# Autodesk Inventor part: 欧标 2020铝合金钢材-01
Saved by Autodesk Inventor 2021 (Build 250183000, 183)
## iProperties
Created: 2025-04-16
Part Number: 欧标 2020铝合金钢材-01
Material: 常规
Document SubType Name: Modeling
Designer: 86155
Standards Organization: GB
Language: zh-CN
Size Designation: 欧标 2020铝合金钢材-01
Categories: <MemberInstance><Categories><Category DisplayName="结构型材" InternalName="089c4875-fa83-4c05-b084-43b9cc11f5ed" Mnemonic="GRDR"><CategoryParameter DisplayName="每单位长度的质量" InternalName="0bb95a10-148f-4027-a459-38d7b056702a" Mnemonic="shpmass"/><CategoryParameter DisplayName="截面面积" InternalName="1ff91680-64b0-4202-b9a3-7fd3f94bba3b" Mnemonic="secarea"/><CategoryParameter DisplayName="旋转半径 (x)" InternalName="25778675-03e9-40c1-b6a8-4a9ed693320d" Mnemonic="gyrradx"/><CategoryParameter DisplayName="扭转刚性模数" InternalName="26c1ec35-5026-4c63-ad0a-751cf684a536" Mnemonic="torrigmod"/><CategoryParameter DisplayName="重心到 X-X 的距离" InternalName="26c9bdb8-9c79-4b4f-a92e-8e197583c9c4" Mnemonic="grcendistX"/><CategoryParameter DisplayName="旧成员 ID" InternalName="340afe4f-75d7-48d3-ab7d-943f3c3da468" Mnemonic="LegacyMemberID"/><CategoryParameter DisplayName="基本长度" InternalName="42e34263-8f20-4d0e-ad48-bf1385b87c24" Mnemonic="shplen"/><CategoryParameter DisplayName="转动惯量 (y)" InternalName="4b9f58ea-bced-460e-81ea-3d29ca5a49e3" Mnemonic="inermomy"/><CategoryParameter DisplayName="转动惯量 (x)" InternalName="4cd780bc-73d7-43ac-917a-579e5cbd684d" Mnemonic="inermomx"/><CategoryParameter DisplayName="自定义基点" InternalName="4f1d1b73-316d-484b-a3df-9cbabb16eb77" Mnemonic="shpBasePoint"/><CategoryParameter DisplayName="形状高度" InternalName="50274e7d-5ac0-4796-92cb-c59e54983c67" Mnemonic="shpheig"/><CategoryParameter DisplayName="截面模数 (y)" InternalName="59eaa5e9-d227-48dc-b6c1-6920f96e0f95" Mnemonic="secmody"/><CategoryParameter DisplayName="截面指示" InternalName="5a64d034-428d-49c8-ba32-7619764de20f" Mnemonic="shpdes"/><CategoryParameter DisplayName="截面模数 (x)" InternalName="72cfad18-cf51-4ed4-aaa7-c6b224f8419f" Mnemonic="secmodx"/><CategoryParameter DisplayName="扭转截面模数" InternalName="7c55a8dc-8844-49f9-a867-cc677b30ec9a" Mnemonic="torsecmod"/><CategoryParameter DisplayName="形状宽度" InternalName="7c717d54-a18f-4666-b4d4-573cce22c62c" Mnemonic="shpwdth"/><CategoryParameter DisplayName="第二个形状厚度" InternalName="9251a8e1-85fd-4e47-af99-afdb762317d9" Mnemonic="shpthick2"/><CategoryParameter DisplayName="编写的 FG" InternalName="9c666724-f362-4ea7-ac62-f6a007de5c69" Mnemonic="shpFGAuto"/><CategoryParameter DisplayName="重心到 Y-Y 的距离" InternalName="bcc4fb17-7af4-436a-8f8c-d0aa3b0248c5" Mnemonic="grcendistY"/><CategoryParameter DisplayName="旋转半径 (y)" InternalName="bfa18ebe-1636-4dbe-8d42-b263e0b73184" Mnemonic="gyrrady"/><CategoryParameter DisplayName="形状厚度" InternalName="d109cf76-8eb4-42fc-9800-4409734adc67" Mnemonic="shpthick"/><CategoryParameter DisplayName="剪切位移系数" InternalName="de4c90c6-aaa8-468f-a335-6737b311b5d3" Mnemonic="shdispc"/><Category DisplayName="其他" InternalName="f02205ff-2390-476f-921c-0b3185f88e84" Mnemonic="OTHSHP"><CategoryParameter DisplayName="转动惯量 (y)" InternalName="044c654e-f649-48ac-84cc-650a29ae31ca" Mnemonic="inermomy"/><CategoryParameter DisplayName="形状厚度" InternalName="12b1a788-9233-48fd-a933-2df8ff42b15f" Mnemonic="shpthick"/><CategoryParameter DisplayName="每单位长度的质量" InternalName="2fd289d6-9394-4d2d-97e6-6659d7d4551d" Mnemonic="shpmass"/><CategoryParameter DisplayName="旋转半径 (y)" InternalName="743e1dfe-1bba-408b-b985-cf752b207386" Mnemonic="gyrrady"/><CategoryParameter DisplayName="截面模数 (y)" InternalName="88b8bff9-a616-4028-93d5-ed4f79680d13" Mnemonic="secmody"/><CategoryParameter DisplayName="截面面积" InternalName="c46ecdf8-b6eb-4db9-8b25-30258930c1e3" Mnemonic="secarea"/><CategoryParameter DisplayName="截面模数 (x)" InternalName="cac70804-9d39-43bb-be17-56ea1f39a6c2" Mnemonic="secmodx"/><CategoryParameter DisplayName="转动惯量 (x)" InternalName="ec6737bc-264f-43ed-b0bd-f6d410c2718d" Mnemonic="inermomx"/><CategoryParameter DisplayName="旋转半径 (x)" InternalName="ee72c61e-565e-4fd6-b448-66e1e1abcb7e" Mnemonic="gyrradx"/></Category></Category><Category DisplayName="数据类型" InternalName="23b78d0f-2648-40c6-8793-ca6db495c9e8" Mnemonic="DATATYPE"><CategoryParameter DisplayName="显示名" InternalName="05415f3d-3907-474b-a020-eb9d644f4cf3" Mnemonic="DISPLAYNAME"/><CategoryParameter DisplayName="标准" InternalName="0c0a119c-1e12-4c84-803f-101930972f5e" Mnemonic="STANDARD"/><CategoryParameter DisplayName="描述" InternalName="13903e3d-64b1-4950-80da-f627842ea37f" Mnemonic="DESCRIPTION"/><CategoryParameter DisplayName="规格" InternalName="2675968c-4ce5-49e0-a4f5-552d29089031" Mnemonic="DESIGNATION"/><CategoryParameter DisplayName="默认列" InternalName="2af9ec52-faaa-4026-b378-f9fa4afca842" Mnemonic="DEFAULTROW"/><CategoryParameter DisplayName="文件夹名称" InternalName="3f06958e-8713-4116-9be7-ed6184ecc97b" Mnemonic="FOLDERNAME"/><CategoryParameter DisplayName="版本指南" InternalName="45a75005-10b1-4dfc-8d6d-dfe629f0b93c" Mnemonic="REVISIONGUID"/><CategoryParameter DisplayName="文件名" InternalName="8b46a4cc-9585-4fed-90c3-899f57e09a73" Mnemonic="FILENAME"/><CategoryParameter DisplayName="标准组织" InternalName="8f5914e1-4693-403f-8ab5-d37768198c9d" Mnemonic="STDSORG"/><CategoryParameter DisplayName="系列版本" InternalName="914462f6-6e19-4b14-ba84-155b9680b1d0" Mnemonic="FAMILYREVISION"/><CategoryParameter DisplayName="标准版本" InternalName="91d5a463-65c2-4fde-b823-3b7fea5e8e17" Mnemonic="STANDARDREVISION"/><CategoryParameter DisplayName="成员版本" InternalName="a65d44b9-392f-4f4f-857b-e4b3d54996fe" Mnemonic="MEMBERREVISION"/><CategoryParameter DisplayName="剪裁格式" InternalName="bc51e27b-3422-4e78-93ef-cec197ddf230" Mnemonic="CLIPFORMAT"/><CategoryParameter DisplayName="制造商" InternalName="cd6c7a72-a28a-4e50-99a9-2c7f4e13e5ad" Mnemonic="MANUFACTURER"/><CategoryParameter DisplayName="内部名称" InternalName="cf1d0246-76d9-4b4a-8305-fa0409afb5c1" Mnemonic="INTERNALNAME"/><CategoryParameter DisplayName="是否公制" InternalName="e2385c5b-1ea4-4823-96a8-8de651266ec3" Mnemonic="ISMETRIC"/><Category DisplayName="零件" InternalName="c0e0b642-3bcb-4cc8-9e80-f96d35c4afa4" Mnemonic="PART"><CategoryParameter DisplayName="零件代号" InternalName="016b6077-bfbe-49bd-92c9-d8d59c39c941" Mnemonic="PARTNUMBER"/><CategoryParameter DisplayName="库存编号" InternalName="4dba7c1c-e26c-444e-836c-b08b433409a8" Mnemonic="STOCKNUMBER"/><CategoryParameter DisplayName="材料键" InternalName="5c9a8adb-dd2b-4535-b97f-0a94a95fe41f" Mnemonic="MATERIALKEY"/><CategoryParameter DisplayName="材料" InternalName="818a152a-d3c3-49ca-80ee-df7d91421b8e" Mnemonic="MATERIAL"/></Category></Category></Categories><FamilyTemplate Id="欧标 2020铝合金钢材"><FamilyTemplateParameters><FamilyTemplateParameter ObjectType="kUserParameterObject" ValueType="xs:double" Id="2" ObjectReferenceKey="圆角"/><FamilyTemplateParameter ObjectType="kUserParameterObject" ValueType="xs:double" Id="3" ObjectReferenceKey="宽度"/><FamilyTemplateParameter ObjectType="kUserParameterObject" ValueType="xs:double" Id="4" ObjectReferenceKey="长度"/><FamilyTemplateParameter ObjectType="kPartComponentDefinitionObject" ValueType="xs:string" Id="6" SubObjectId="Material"/><FamilyTemplateParameter ObjectType="kPropertyObject" ValueType="xs:string" Id="18" ObjectReferenceKey="{32853F0F-3444-11d1-9E93-0060B03C1CA6}" SubObjectId="5"/><FamilyTemplateParameter ObjectType="kPropertyObject" ValueType="xs:string" Id="19" ObjectReferenceKey="{32853F0F-3444-11d1-9E93-0060B03C1CA6}" SubObjectId="52"/></FamilyTemplateParameters></FamilyTemplate><CategoryParameterMap><ParamToTemplateMap><ParamToTemplate CategoryParameter="//CategoryParameter[@InternalName='cf1d0246-76d9-4b4a-8305-fa0409afb5c1']" ConstantValue="f6263a19-3060-40e9-a912-404bc1cf63e0"/><ParamToTemplate CategoryParameter="//CategoryParameter[@InternalName='45a75005-10b1-4dfc-8d6d-dfe629f0b93c']" ConstantValue="6f9f3c90-dcaa-4261-b2d0-a83ec9cae418"/><ParamToTemplate CategoryParameter="//CategoryParameter[@InternalName='3f06958e-8713-4116-9be7-ed6184ecc97b']" ConstantValue="欧标 2020铝合金钢材"/><ParamToTemplate CategoryParameter="//CategoryParameter[@InternalName='8f5914e1-4693-403f-8ab5-d37768198c9d']" ConstantValue="GB"/><ParamToTemplate CategoryParameter="//CategoryParameter[@InternalName='0c0a119c-1e12-4c84-803f-101930972f5e']" TemplateParameter="12"/><ParamToTemplate CategoryParameter="//CategoryParameter[@InternalName='91d5a463-65c2-4fde-b823-3b7fea5e8e17']" TemplateParameter="13"/><ParamToTemplate CategoryParameter="//CategoryParameter[@InternalName='cd6c7a72-a28a-4e50-99a9-2c7f4e13e5ad']" TemplateParameter="14"/><ParamToTemplate CategoryParameter="//CategoryParameter[@InternalName='13903e3d-64b1-4950-80da-f627842ea37f']" TemplateParameter="15"/><ParamToTemplate CategoryParameter="//CategoryParameter[@InternalName='05415f3d-3907-474b-a020-eb9d644f4cf3']" ConstantValue="欧标 2020铝合金钢材"/><ParamToTemplate CategoryParameter="//CategoryParameter[@InternalName='914462f6-6e19-4b14-ba84-155b9680b1d0']" ConstantValue="11"/><ParamToTemplate CategoryParameter="//CategoryParameter[@InternalName='bc51e27b-3422-4e78-93ef-cec197ddf230']" ConstantValue="CF_INVENTOR.STDPARTS"/><ParamToTemplate CategoryParameter="//CategoryParameter[@InternalName='e2385c5b-1ea4-4823-96a8-8de651266ec3']" ConstantValue="true"/><ParamToTemplate CategoryParameter="//CategoryParameter[@InternalName='2af9ec52-faaa-4026-b378-f9fa4afca842']" ConstantValue="1"/><ParamToTemplate CategoryParameter="//CategoryParameter[@InternalName='9c666724-f362-4ea7-ac62-f6a007de5c69']" ConstantValue="1"/><ParamToTemplate CategoryParameter="//CategoryParameter[@InternalName='8b46a4cc-9585-4fed-90c3-899f57e09a73']" ConstantValue="欧标 2020铝合金钢材-01"/><ParamToTemplate CategoryParameter="//CategoryParameter[@InternalName='a65d44b9-392f-4f4f-857b-e4b3d54996fe']" ConstantValue="6a432091-89bb-4127-b7c1-9c8b6e7916ae"/><ParamToTemplate CategoryParameter="//CategoryParameter[@InternalName='a65d44b9-392f-4f4f-857b-e4b3d54996fe']" ConstantValue="6a432091-89bb-4127-b7c1-9c8b6e7916ae"/><ParamToTemplate CategoryParameter="//CategoryParameter[@InternalName='2675968c-4ce5-49e0-a4f5-552d29089031']" TemplateParameter="19"/><ParamToTemplate CategoryParameter="//CategoryParameter[@InternalName='818a152a-d3c3-49ca-80ee-df7d91421b8e']" TemplateParameter="6"/><ParamToTemplate CategoryParameter="//CategoryParameter[@InternalName='016b6077-bfbe-49bd-92c9-d8d59c39c941']" TemplateParameter="18"/><ParamToTemplate CategoryParameter="//CategoryParameter[@InternalName='42e34263-8f20-4d0e-ad48-bf1385b87c24']" TemplateParameter="4"/></ParamToTemplateMap></CategoryParameterMap></MemberInstance>
Density: 1 g/cm^3
Appearance: 默认
_CCFamilyMember: 1
_CCFamilyDisplayName: 欧标 2020铝合金钢材
_FrameMemberDoc: Frame Member File
_Version: 25.0.0
_GetPNFromCC: 1
G_L: 910.000 mm
G_W: 20.000 mm
G_H: 20.000 mm
+0E0289C9-3460-4F08-99CE-0A15E25D59BD+切割明细1: 交角 90.00 deg
IsCustomPart: 1
Author: 86155
Autodesk Inventor part; units mm, degrees
ref_plane "起始平面" through (0, -10, 0) normal (0, 1, 0) x (-1, 0, 0)
ref_plane "终止平面" through (0, 900, 0) normal (0, 1, 0) x (-1, 0, 0)
sketch "草图" plane through (0, 0, 0) normal (0, 1, 0) x (-1, 0, 0)
  line L0 (-9.1, 10.0192) -> (-9.101, 10.0203)
  line L1 (-10, 10) -> (-9.5607, 9.5607) construction
  arc A0 (-8.5, 10) -> (-10, 8.5) centre (-8.5, 8.5) ccw
  circle A1 centre (0, 0) radius 2.5
  line L2 (-2.9808, 3.9) -> (0, 3.9)
  line L3 (-3.9, 0) -> (-3.9, 2.9808)
  line L4 (-2.5, 0) -> (-3.1, 0)
  line L5 (2.9808, 3.9) -> (0, 3.9)
  circle A2 centre (0, 0) radius 2.5
  circle A3 centre (0, 0) radius 2.5
  circle A4 centre (0, 0) radius 2.5
  line L6 (0, 16.3557) -> (0, -12.0006)
  line L7 (-4.3, 9.1) -> (-4.3, 10)
  line L8 (2.9808, -3.9) -> (0, -3.9)
  line L9 (-3.9, 0) -> (-3.9, -2.9808)
  line L10 (3.9, 0) -> (3.9, -2.9808)
  line L11 (-2.9808, -3.9) -> (-5.5, -6.4192)
  line L12 (-2.9808, -3.9) -> (0, -3.9)
  line L13 (3.8, -8.2) -> (3.8, -9.1)
  line L14 (5.5, -6.4192) -> (2.9808, -3.9)
  line L15 (3.8, -9.1) -> (4.3, -9.1)
  line L16 (5.5, -8.2) -> (3.8, -8.2)
  line L17 (5.5, -8.2) -> (5.5, -6.4192)
  line L18 (3.9, -2.9808) -> (6.4192, -5.5)
  line L19 (8.2, -3.8) -> (8.2, -5.5)
  line L20 (8.2, -5.5) -> (6.4192, -5.5)
  line L21 (8.2, -3.8) -> (9.1, -3.8)
  line L22 (9.1, -3.8) -> (9.1, -4.3)
  line L23 (9.1, -4.3) -> (10, -4.3)
  line L24 (10, -4.3) -> (10, -8.5)
  arc A5 (8.5, -10) -> (10, -8.5) centre (8.5, -8.5) ccw
  line L25 (8.5, -10) -> (4.3, -10)
  line L26 (4.3, -9.1) -> (4.3, -10)
  line L27 (5.5, 6.4192) -> (2.9808, 3.9)
  line L28 (3.9, 2.9808) -> (6.4192, 5.5)
  line L29 (10, 4.3) -> (10, 8.5)
  line L30 (3.9, 0) -> (3.9, 2.9808)
  line L31 (5.5, 8.2) -> (5.5, 6.4192)
  line L32 (5.5, 8.2) -> (3.8, 8.2)
  line L33 (4.3, 9.1) -> (4.3, 10)
  arc A6 (10, 8.5) -> (8.5, 10) centre (8.5, 8.5) ccw
  line L34 (8.5, 10) -> (4.3, 10)
  line L35 (8.2, 3.8) -> (9.1, 3.8)
  line L36 (9.1, 4.3) -> (10, 4.3)
  line L37 (9.1, 3.8) -> (9.1, 4.3)
  line L38 (8.2, 3.8) -> (8.2, 5.5)
  line L39 (8.2, 5.5) -> (6.4192, 5.5)
  line L40 (3.8, 8.2) -> (3.8, 9.1)
  line L41 (3.8, 9.1) -> (4.3, 9.1)
  line L42 (-10, 4.3) -> (-10, 8.5)
  line L43 (-8.5, 10) -> (-4.3, 10)
  line L44 (-9.1, 4.3) -> (-10, 4.3)
  line L45 (-9.1, 3.8) -> (-9.1, 4.3)
  line L46 (-8.2, 3.8) -> (-9.1, 3.8)
  line L47 (-8.2, 5.5) -> (-6.4192, 5.5)
  line L48 (-8.2, 3.8) -> (-8.2, 5.5)
  line L49 (-5.5, 8.2) -> (-5.5, 6.4192)
  line L50 (-3.8, 9.1) -> (-4.3, 9.1)
  line L51 (-3.8, 8.2) -> (-3.8, 9.1)
  line L52 (-5.5, 8.2) -> (-3.8, 8.2)
  line L53 (-3.9, 2.9808) -> (-6.4192, 5.5)
  line L54 (-2.9808, 3.9) -> (-5.5, 6.4192)
  line L55 (-5.5, -8.2) -> (-3.8, -8.2)
  line L56 (-5.5, -8.2) -> (-5.5, -6.4192)
  line L57 (-3.9, -2.9808) -> (-6.4192, -5.5)
  line L58 (-3.8, -8.2) -> (-3.8, -9.1)
  line L59 (-3.8, -9.1) -> (-4.3, -9.1)
  line L60 (-4.3, -9.1) -> (-4.3, -10)
  line L61 (-8.2, -5.5) -> (-6.4192, -5.5)
  line L62 (-8.2, -3.8) -> (-9.1, -3.8)
  line L63 (-9.1, -3.8) -> (-9.1, -4.3)
  line L64 (-8.5, -10) -> (-4.3, -10)
  line L65 (-9.1, -4.3) -> (-10, -4.3)
  line L66 (-10, -4.3) -> (-10, -8.5)
  arc A7 (-10, -8.5) -> (-8.5, -10) centre (-8.5, -8.5) ccw
  line L67 (-8.2, -3.8) -> (-8.2, -5.5)
  dimension "圆角" = 1.5
  dimension "宽度" = 20
  constraints: 136 end point, 18 symmetric about line, 9 point on circle, 6 centre point, 4 coincident, 4 horizontal, 4 perpendicular, 3 point on line, 2 horizontal alignment, 2 tangent, 1 line through centre, 1 parallel, 1 vertical, 5 other
  measures "圆角" radius of A0
  measures "宽度" distance between parallel lines of L43 L64
extrude "实体" add sketch "草图" along normal up to surface (910 mm away) from surface at -10 contours L43 L7 L50 L51 L52 L49 L54 L2 L6 A1 L12 L11 L56 L55 L58 L59 L60 L64 A7 L66 L65 L63 L62 L67 L61 L57 L9 L3 L53 L47 L48 L46 L45 L44 L42 A0 | L5 L27 L31 L32 L40 L41 L33 L34 A6 L29 L36 L37 L35 L38 L39 L28 L30 L10 L18 L20 L19 L21 L22 L23 L24 A5 L25 L26 L15 L13 L16 L17 L14 L8 L6 A1
sketch "草图2" plane through (0, 0, 0) normal (0, 1, 0) x (-1, 0, 0)
  line L0 (0, 0) -> (10, 0)
ref_plane "工作平面3" through (0, 0, 0) normal (0, 0, -1) x (-1, 0, 0)
sketch "草图3" plane through (0, 0, 0) normal (0, 0, -1) x (-1, 0, 0)
  line L0 (-2, -10) -> (12, -10)
  line L1 (-2, 900) -> (12, 900)
  dimension "d11" = 910
  measures "d11" distance between parallel lines of L0 L1
ref_plane "工作平面4" through (4.3, -10, -800) normal (0, -1, 0) x (1, 0, 0)
split "分割1" plane through (4.3, -10, -800) removes the side toward (0, -1, 0)
equation "\"G_OFFSET_END\" = 0"
equation "\"G_L\" = d11"
